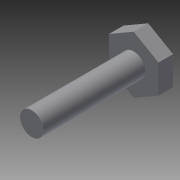
# Autodesk Inventor part: катушка
Saved by Autodesk Inventor 2013 (Build 170138000, 138)
## iProperties
Created: 2014-04-30
Part Number: катушка
Material: Типовые
Document SubType Name: Modeling
Designer: HP1
Density: 1 g/cm^3
Author: HP1
Autodesk Inventor part; units mm, degrees
ref_plane "YZ Plane" through (0, 0, 0) normal (1, 0, 0) x (0, 1, 0)
ref_plane "XZ Plane" through (0, 0, 0) normal (0, 1, 0) x (-1, 0, 0)
ref_plane "XY Plane" through (0, 0, 0) normal (0, 0, 1) x (1, 0, 0)
sketch "Эскиз1" plane through (0, 0, 0) normal (0, 1, 0) x (-1, 0, 0)
  circle A0 centre (0, 0) radius 4
  dimension "d0" = 8
  constraints: 1 centre point
  measures "d0" diameter of A0
extrude "Выдавливание1" add sketch "Эскиз1" along normal blind 35
sketch "Эскиз2" plane through (0, 35, 0) normal (0, 1, 0) x (1, 0, 0)
  circle A0 centre (0, 0) radius 4 projected
  line L0 (8.5, -4.9075) -> (0, -9.815)
  line L1 (0, -9.815) -> (-8.5, -4.9075)
  line L2 (-8.5, -4.9075) -> (-8.5, 4.9075)
  line L3 (-8.5, 4.9075) -> (0, 9.815)
  line L4 (0, 9.815) -> (8.5, 4.9075)
  line L5 (8.5, 4.9075) -> (8.5, -4.9075)
  dimension "d3" = 17
  constraints: 12 end point, 13 other
  measures "d3" distance between parallel lines of L5 L2
extrude "Выдавливание2" add sketch "Эскиз2" along normal blind 5
